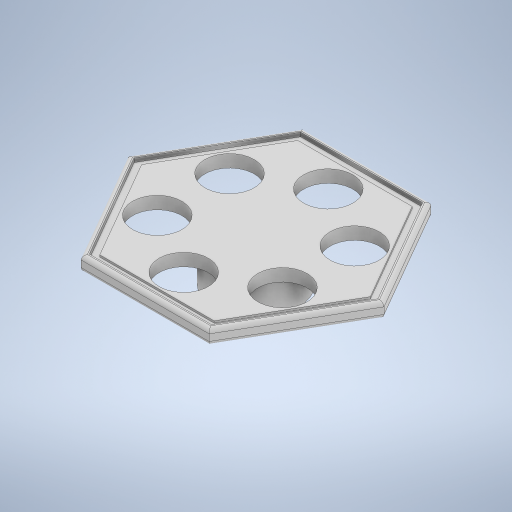
# Autodesk Inventor part: OV-PAM_n_6_bottom
Saved by Autodesk Inventor 2024 (Build 280153000, 153)
## iProperties
Created: 2023-08-31
Part Number: OV-PAM_n_6_bottom
Material: 일반
Document SubType Name: Modeling
Designer: jsw
Density: 1 g/cm^3
Appearance: 기본값
Author: jsw
Autodesk Inventor part; units mm, degrees
ref_plane "YZ Plane" through (0, 0, 0) normal (1, 0, 0) x (0, 1, 0)
ref_plane "XZ Plane" through (0, 0, 0) normal (0, 1, 0) x (-1, 0, 0)
ref_plane "XY Plane" through (0, 0, 0) normal (0, 0, 1) x (1, 0, 0)
sketch "스케치1" plane through (0, 0, 0) normal (0, 1, 0) x (-1, 0, 0)
  line L0 (17.6385, -30.5508) -> (-17.6385, -30.5508)
  line L1 (-17.6385, -30.5508) -> (-35.277, 0)
  line L2 (-35.277, 0) -> (-17.6385, 30.5508)
  line L3 (-17.6385, 30.5508) -> (17.6385, 30.5508)
  line L4 (17.6385, 30.5508) -> (35.277, 0)
  line L5 (35.277, 0) -> (17.6385, -30.5508)
  line L6 (19.486, -33.7508) -> (-19.486, -33.7508)
  line L7 (-19.486, -33.7508) -> (-38.972, 0)
  line L8 (-38.972, 0) -> (-19.486, 33.7508)
  line L9 (-19.486, 33.7508) -> (19.486, 33.7508)
  line L10 (19.486, 33.7508) -> (38.972, 0)
  line L11 (38.972, 0) -> (19.486, -33.7508)
  point P0 (0, 0)
  point P1 (0, 0)
  point P2 (0, 0)
  dimension "d0" = 70.554
  dimension "d1" = 3.2
  constraints: 24 end point, 2 coincident, 2 horizontal, 26 other
  measures "d0" distance of L2.end L0.start
  measures "d1" distance between parallel lines of L0 L6
extrude "돌출1" add sketch "스케치1" along normal blind 4.4 contours L0 L1 L2 L3 L4 L5 | L6 L7 L8 L9 L10 L11
sketch "스케치2" plane through (0, 4.4, 0) normal (0, 1, 0) x (1, 0, 0)
  line L0 (-18.5623, 32.1508) -> (18.5623, 32.1508)
  line L1 (18.5623, 32.1508) -> (37.1245, 0)
  line L2 (37.1245, 0) -> (18.5623, -32.1508)
  line L3 (18.5623, -32.1508) -> (-18.5623, -32.1508)
  line L4 (-18.5623, -32.1508) -> (-37.1245, 0)
  line L5 (-37.1245, 0) -> (-18.5623, 32.1508)
  line L6 (-19.486, 33.7508) -> (-38.972, 0) projected
  point P0 (0, 0)
  point P1 (0, 0)
  dimension "d4" = 1.6
  constraints: 12 end point, 1 coincident, 1 horizontal, 13 other
  measures "d4" distance between parallel lines of L5 L6
extrude "돌출2" cut sketch "스케치2" against normal blind 1.2
sketch "스케치3" plane through (0, 3.2, 0) normal (0, 1, 0) x (1, 0, 0)
  line L0 (17.4076, -30.1508) -> (-17.4076, -30.1508)
  line L1 (-17.4076, -30.1508) -> (-34.8151, 0)
  line L2 (-34.8151, 0) -> (-17.4076, 30.1508)
  line L3 (-17.4076, 30.1508) -> (17.4076, 30.1508)
  line L4 (17.4076, 30.1508) -> (34.8151, 0)
  line L5 (34.8151, 0) -> (17.4076, -30.1508)
  line L6 (-18.5623, 32.1508) -> (18.5623, 32.1508) projected
  point P0 (0, 0)
  point P1 (0, 0)
  dimension "d7" = 2
  constraints: 12 end point, 1 coincident, 1 horizontal, 13 other
  measures "d7" distance between parallel lines of L6 L3
extrude "돌출3" add sketch "스케치3" along normal blind 0.6
fillet "모깎기1" radius 1.2 12 edges at (0, 4.4, -33.7508) (0, 0, -33.7508) (-29.229, 4.4, -16.8754) (-29.229, 0, -16.8754) (-29.229, 4.4, 16.8754) (-29.229, 0, 16.8754) (0, 0, 33.7508) (0, 4.4, 33.7508) (29.229, 0, 16.8754) (29.229, 4.4, 16.8754) (29.229, 4.4, -16.8754) (29.229, 0, -16.8754)
sketch "스케치11" plane through (0, 0, 0) normal (0, -1, 0) x (1, 0, 0)
  circle A0 centre (0, 0) radius 12.7
  dimension "d49" = 25.4
  constraints: 1 centre point, 1 coincident
  measures "d49" diameter of A0
extrude "돌출11" add sketch "스케치11" along normal blind 10.16
sketch "스케치12" plane through (0, -10.16, 0) normal (0, -1, 0) x (1, 0, 0)
  circle A0 centre (0, 0) radius 4.5
  line L0 (-2.5981, 4.5) -> (2.5981, 4.5)
  line L1 (2.5981, 4.5) -> (5.1962, 0)
  line L2 (5.1962, 0) -> (2.5981, -4.5)
  line L3 (2.5981, -4.5) -> (-2.5981, -4.5)
  line L4 (-2.5981, -4.5) -> (-5.1962, 0)
  line L5 (-5.1962, 0) -> (-2.5981, 4.5)
  point P0 (-3.8971, 2.25)
  point P1 (-3.8971, -2.25)
  point P2 (0, 4.5)
  point P3 (0, -4.5)
  point P4 (3.8971, -2.25)
  point P5 (3.8971, 2.25)
  dimension "d52" = 9
  constraints: 12 end point, 2 coincident, 1 centre point, 1 horizontal, 1 tangent, 13 other
  measures "d52" diameter of A0
extrude "돌출12" cut sketch "스케치12" against normal blind 12
sketch "스케치13" plane through (0, 0, 0) normal (0, -1, 0) x (1, 0, 0)
  circle A0 centre (0, -22) radius 7.5
  circle A1 centre (19.0526, -11) radius 7.5
  circle A2 centre (19.0526, 11) radius 7.5
  circle A3 centre (0, 22) radius 7.5
  circle A4 centre (-19.0526, 11) radius 7.5
  circle A5 centre (-19.0526, -11) radius 7.5
  point P0 (0, 0)
  dimension "d57" = 15
  dimension "d58" = 22
  dimension "d61" = 360
  constraints: 6 centre point, 1 vertical alignment, 13 other
  measures "d57" diameter of A0
  measures "d58" distance of A0.centre point (0, 0)
extrude "돌출13" cut sketch "스케치13" against normal up to surface (3.8 mm away)
sketch "스케치16" plane through (0, 1.84, 0) normal (0, -1, 0) x (1, 0, 0)
  line L0 (-2.5981, 4.5) -> (2.5981, 4.5) projected
  line L1 (-5.1962, 0) -> (-2.5981, 4.5) projected
  line L2 (-2.5981, -4.5) -> (-5.1962, 0) projected
  line L3 (2.5981, -4.5) -> (-2.5981, -4.5) projected
  line L4 (5.1962, 0) -> (2.5981, -4.5) projected
  line L5 (2.5981, 4.5) -> (5.1962, 0) projected
  line L6 (-2.0207, 3.5) -> (2.0207, 3.5)
  line L7 (2.0207, 3.5) -> (4.0415, 0)
  line L8 (4.0415, 0) -> (2.0207, -3.5)
  line L9 (2.0207, -3.5) -> (-2.0207, -3.5)
  line L10 (-2.0207, -3.5) -> (-4.0415, 0)
  line L11 (-4.0415, 0) -> (-2.0207, 3.5)
  point P0 (0, 0)
  point P1 (0, 0)
  point P2 (0, 3.5)
  dimension "d83" = 1
  constraints: 12 end point, 1 coincident, 1 horizontal, 1 midpoint, 13 other
  measures "d83" distance between parallel lines of L6 L0
extrude "돌출14" add sketch "스케치16" along normal blind 8.5
fillet "모깎기2" radius 0.5 6 edges at (0, -10.16, 4.5) (-3.8971, -10.16, 2.25) (3.8971, -10.16, 2.25) (3.8971, -10.16, -2.25) (-3.8971, -10.16, -2.25) (0, -10.16, -4.5)
equation "\"d72\" = 55deg"
